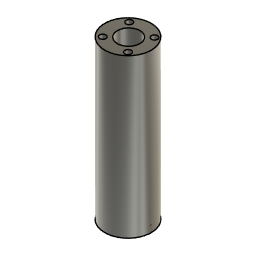
wand hilt 2 (Autodesk Fusion 360 design; units mm, degrees)
part number: 2025-05-15-15-05-41-209
Autodesk Fusion 360 part; units mm, degrees
sketch "Sketch1" plane through (0, 0, 0) normal (0, 0, 1) x (1, 0, 0)
  circle A0 centre (0, 0) radius 17.5
  line L0 (-10, 13) -> (10, 13)
  line L1 (10, 13) -> (10, -13)
  line L2 (10, -13) -> (-10, -13)
  line L3 (-10, -13) -> (-10, 13)
  dimension "d1" = 35
  dimension "d2" = 20
  dimension "d3" = 26
  dimension "d4" = 13
  dimension "d5" = 10
  constraint coincident A0.centre origin
  constraint horizontal L0
  constraint vertical L1
  constraint horizontal L2
  constraint vertical L3
  measures "d1" diameter of A0
  measures "d2" distance of L0.start L0.end
  measures "d3" distance of L0.start L2.end
  measures "d4" distance of A0.centre L0
  measures "d5" distance of A0.centre L1
extrude "Extrude1" add sketch "Sketch1" along normal blind 65
sketch "Sketch2" plane through (0, 0, 65) normal (0, 0, 1) x (-1, 0, 0)
  line L0 (-10, 13) -> (10, 13)
  line L1 (10, 13) -> (10, -13)
  line L2 (10, -13) -> (-10, -13)
  line L3 (-10, -13) -> (-10, 13)
  circle A0 centre (0, 0) radius 17.5
  circle A1 centre (0, 0) radius 17.5
  circle A2 centre (-0.4739, 0) radius 5
  dimension "d8" = 10
  constraint concentric A0 A1
  measures "d8" diameter of A2
extrude "Extrude2" add sketch "Sketch2" along normal blind 2 contours L0 L1 L2 L3 | A0 A1
sketch "Sketch3" plane through (0, 0, 67) normal (0, 0, 1) x (-1, 0, 0)
  circle A0 centre (-0.4739, 0) radius 5
  circle A1 centre (0, 0) radius 17.5
  circle A2 centre (-0.4739, 0) radius 8.5
  dimension "d11" = 17
  constraint concentric A0 A2
  measures "d11" diameter of A2
extrude "Extrude3" add sketch "Sketch3" along normal blind 52 contours A1
fillet "Fillet1" radius 3 1 edges at (8.3987, 3.0737, 67)
form "Form1" [no effect]
sketch "Sketch4" plane through (0, 0, 0) normal (0, 0, 1) x (1, 0, 0)
  circle A0 centre (-15, 0) radius 2
  circle A1 centre (0, 0) radius 17.5
  circle A2 centre (15, 0) radius 2
  dimension "d16" = 4
  dimension "d17" = 15
  dimension "d18" = 4
  dimension "d19" = 15
  measures "d16" diameter of A0
  measures "d17" distance of A0.centre A1.centre
  measures "d18" diameter of A2
  measures "d19" distance of A2.centre A1.centre
extrude "Extrude4" cut sketch "Sketch4" along normal blind 5 contours A0 | A2
sketch "Sketch5" plane through (0, 0, 119) normal (0, 0, 1) x (-1, 0, 0)
  circle A0 centre (-0.4739, 0) radius 8.5
  circle A1 centre (0, 0) radius 17.5
  circle A2 centre (-10, 10) radius 2.4
  circle A3 centre (9.5261, 9.5261) radius 2.4
  circle A4 centre (9.0522, -10) radius 2.4
  circle A5 centre (-10.4739, -9.5261) radius 2.4
  point P0 (-10.4739, -9.5261)
  point P1 (9.0522, -10)
  point P2 (9.5261, 9.5261)
  dimension "d22" = 4.8
  dimension "d24" = 10
  dimension "d26" = 360
  dimension "d27" = 4.8
  dimension "d28" = 4.8
  dimension "d29" = 4.8
  constraint coincident P2 A3.centre
  constraint coincident P1 A4.centre
  constraint coincident P0 A5.centre
  measures "d22" diameter of A2
  measures "d24" vertical distance of A1.centre A2.centre
  measures "d27" diameter of A3
  measures "d28" diameter of A4
  measures "d29" diameter of A5
extrude "Extrude5" add sketch "Sketch5" along normal blind 4 contours A2 | A3 | A4 | A5
extrude "Extrude6" cut 4 faces at (-7.9226, -10.0912, 123) (-9.2144, 9.325, 123) (10.3117, 8.8511, 123) (8.3101, -9.8134, 123) along direction (0, 0, -1) blind 10
